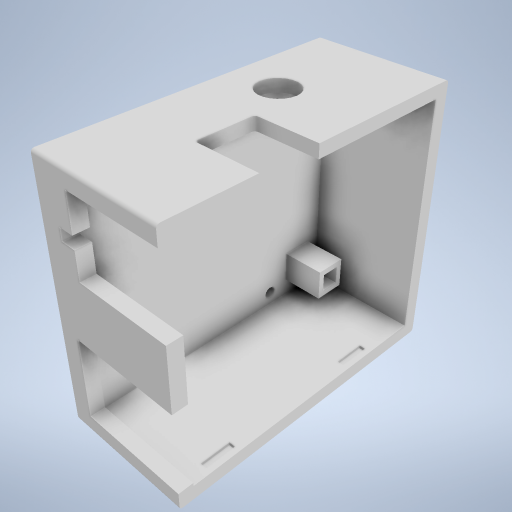
# Autodesk Inventor part: Enclosure_Top_v2
Saved by Autodesk Inventor 2023 (Build 270158030, 158C)
## iProperties
Created: 2023-12-07
Part Number: Enclosure_Top_v2
Material: Generic
Document SubType Name: Sheet Metal
Designer: Fabian
Density: 1 g/cm^3
Sheet Metal Rule: Default_mm
Appearance: Default
Author: Fabian
Autodesk Inventor part; units mm, degrees
ref_plane "YZ Plane" through (0, 0, 0) normal (1, 0, 0) x (0, 1, 0)
ref_plane "XZ Plane" through (0, 0, 0) normal (0, 1, 0) x (-1, 0, 0)
ref_plane "XY Plane" through (0, 0, 0) normal (0, 0, 1) x (1, 0, 0)
sketch "Sketch1" plane through (0, 0, 0) normal (1, 0, 0) x (0, 1, 0)
  line L0 (10.2141, 17.9541) -> (-31.7859, 17.9541)
  line L1 (-31.7859, 17.9541) -> (-31.7859, -30.1559)
  line L2 (-31.7859, -30.1559) -> (10.2141, -30.1559)
  line L3 (10.2141, -30.1559) -> (10.2141, 17.9541)
  point P0 (0, 0)
  dimension "d0" = 42
  dimension "d1" = 48.11
  constraints: 8 end point, 2 parallel, 1 horizontal, 1 perpendicular
  measures "d0" distance of L2.end L1.end
  measures "d1" distance of L1.end L0.end
extrude "BasePlate" add sketch "Sketch1" along normal blind 3
sketch "Sketch2" plane through (3, 0, 0) normal (1, 0, 0) x (0, 0, -1)
  point P0 (0, 0)
sketch "Sketch3" plane through (3, 0, 0) normal (1, 0, 0) x (0, 0, -1)
  line L0 (30.1559, 10.2141) -> (-17.9541, 10.2141) projected
  line L1 (-17.9541, -31.7859) -> (30.1559, -31.7859) projected
  line L2 (-17.9541, 10.2141) -> (30.1559, 10.2141)
  line L3 (30.1559, 10.2141) -> (30.1559, -31.7859)
  line L4 (30.1559, -31.7859) -> (-17.9541, -31.7859)
  line L5 (-17.9541, -31.7859) -> (-17.9541, 10.2141)
  line L6 (-15.5541, 8.2141) -> (27.7559, 8.2141)
  line L7 (27.7559, 8.2141) -> (27.7559, -29.3859)
  line L8 (27.7559, -29.3859) -> (-15.5541, -29.3859)
  line L9 (-15.5541, -29.3859) -> (-15.5541, 8.2141)
  point P0 (0, 0)
  point P1 (-17.9541, -10.7859)
  dimension "d4" = 2
  dimension "d5" = 2.4
  dimension "d6" = 2.4
  dimension "d7" = 2.4
  constraints: 16 end point, 4 parallel, 2 horizontal, 2 perpendicular, 1 midpoint
  measures "d4" distance between parallel lines of L0 L6
  measures "d5" distance between parallel lines of L1 L8
  measures "d6" distance from line of point (-17.954, -10.786) L9
  measures "d7" distance between parallel lines of L3 L7
extrude "Walls" add sketch "Sketch3" along normal blind 18.5
sketch "Sketch4" plane through (21.5, 0, 0) normal (1, 0, 0) x (0, 0, -1)
  line L0 (30.1559, 10.2141) -> (-17.9541, 10.2141) projected
  line L1 (-15.5541, 8.2141) -> (27.7559, 8.2141) projected
  line L2 (-4.1541, 10.2141) -> (5.2459, 10.2141)
  line L3 (5.2459, 10.2141) -> (5.2459, 8.2141)
  line L4 (5.2459, 8.2141) -> (-4.1541, 8.2141)
  line L5 (-4.1541, 8.2141) -> (-4.1541, 10.2141)
  line L6 (-17.9541, 10.2141) -> (-17.9541, -31.7859) projected
  point P0 (0, 0)
  point P1 (-4.1541, 9.2141)
  point P2 (5.2459, 10.2141)
  dimension "d10" = 9.4
  dimension "d11" = 13.8
  constraints: 8 end point, 2 parallel, 2 point on line, 1 horizontal, 1 midpoint, 1 perpendicular
  measures "d10" distance of L3.end L4.end
  measures "d11" distance from line of point (-4.154, 9.214) L6
extrude "USB-C" cut sketch "Sketch4" against normal blind 10.1
sketch "Sketch5" plane through (21.5, 0, 0) normal (1, 0, 0) x (0, 0, -1)
  line L0 (-17.9541, 10.2141) -> (-17.9541, -31.7859) projected
  line L1 (-15.5541, -29.3859) -> (-15.5541, 8.2141) projected
  line L2 (-17.9541, -4.8859) -> (-15.5541, -4.8859)
  line L3 (-15.5541, -4.8859) -> (-15.5541, 7.5141)
  line L4 (-15.5541, 7.5141) -> (-17.9541, 7.5141)
  line L5 (-17.9541, 7.5141) -> (-17.9541, -4.8859)
  line L6 (-4.1541, 10.2141) -> (-17.9541, 10.2141) projected
  point P0 (0, 0)
  point P1 (-16.7541, 7.5141)
  point P2 (-17.9541, 7.5141)
  point P3 (-15.5541, -4.8859)
  dimension "d14" = 12.4
  dimension "d15" = 2.7
  constraints: 8 end point, 2 parallel, 2 point on line, 1 horizontal, 1 midpoint, 1 perpendicular
  measures "d14" distance of L3.end L2.end
  measures "d15" distance from line of L6 point (-16.754, 7.514)
extrude "PowerConnector1" cut sketch "Sketch5" against normal blind 15.5
sketch "Sketch6" plane through (6, 0, 0) normal (1, 0, 0) x (0, 0, -1)
  line L0 (-17.9541, 10.2141) -> (-17.9541, -31.7859) projected
  line L1 (-17.9541, -0.3859) -> (-15.5541, -0.3859)
  line L2 (-15.5541, -0.3859) -> (-15.5541, 1.6141)
  line L3 (-15.5541, 1.6141) -> (-17.9541, 1.6141)
  line L4 (-17.9541, 1.6141) -> (-17.9541, -0.3859)
  line L5 (-17.9541, 7.5141) -> (-15.5541, 7.5141) projected
  point P0 (0, 0)
  dimension "d18" = 2.4
  dimension "d19" = 2
  dimension "d20" = 5.9
  constraints: 8 end point, 2 parallel, 1 horizontal, 1 perpendicular, 1 point on line
  measures "d18" distance of L3.end L2.end
  measures "d19" distance of L1.end L2.end
  measures "d20" distance between parallel lines of L5 L3
extrude "PowerConnector2" cut sketch "Sketch6" against normal blind 2.5
sketch "Sketch8" plane through (21.5, 0, 0) normal (1, 0, 0) x (0, 0, -1)
  line L0 (-17.9541, 10.2141) -> (-17.9541, -31.7859) projected
  line L1 (-15.5541, 8.2141) -> (-15.5541, -29.3859) projected
  line L2 (-17.9541, -28.7859) -> (-15.5541, -28.7859)
  line L3 (-15.5541, -28.7859) -> (-15.5541, -15.1859)
  line L4 (-15.5541, -15.1859) -> (-17.9541, -15.1859)
  line L5 (-17.9541, -15.1859) -> (-17.9541, -28.7859)
  line L6 (-17.9541, -31.7859) -> (30.1559, -31.7859) projected
  point P0 (0, 0)
  dimension "d23" = 13.6
  dimension "d24" = 3
  constraints: 8 end point, 2 parallel, 2 point on line, 1 horizontal, 1 perpendicular
  measures "d23" distance of L3.end L2.end
  measures "d24" distance between parallel lines of L6 L2
extrude "RJ-12" cut sketch "Sketch8" against normal blind 18.1
fillet "Fillet1" radius 0.5 4 edges at (10.75, 10.2141, 17.9541) (10.75, -31.7859, 17.9541) (10.75, 10.2141, -30.1559) (10.75, -31.7859, -30.1559)
sketch "Sketch9" plane through (0, 0, 0) normal (-1, 0, 0) x (0, 0, 1)
  line L0 (-24.5559, -25.4859) -> (-21.5559, -25.4859)
  line L1 (-21.5559, -25.4859) -> (-21.5559, -22.4859)
  line L2 (-21.5559, -22.4859) -> (-24.5559, -22.4859)
  line L3 (-24.5559, -22.4859) -> (-24.5559, -25.4859)
  line L4 (-30.1559, -31.2859) -> (-30.1559, 9.7141) projected
  line L5 (17.4541, -31.7859) -> (-29.6559, -31.7859) projected
  point P0 (0, 0)
  point P1 (-24.5559, -23.9859)
  dimension "d28" = 3
  dimension "d29" = 3
  dimension "d30" = 5.6
  dimension "d31" = 6.3
  constraints: 8 end point, 2 parallel, 1 horizontal, 1 midpoint, 1 perpendicular
  measures "d28" distance of L2.end L1.end
  measures "d29" distance of L1.end L0.end
  measures "d30" distance from line of L4 point (-24.556, -23.986)
  measures "d31" distance between parallel lines of L5 L0
extrude "ZBButton" cut sketch "Sketch9" against normal blind 3
sketch "Sketch10" plane through (0, 0, 0) normal (-1, 0, 0) x (0, 0, 1)
  line L0 (-24.5559, 0.9141) -> (-21.5559, 0.9141)
  line L1 (-21.5559, 0.9141) -> (-21.5559, 3.9141)
  line L2 (-21.5559, 3.9141) -> (-24.5559, 3.9141)
  line L3 (-24.5559, 3.9141) -> (-24.5559, 0.9141)
  line L4 (-30.1559, -31.2859) -> (-30.1559, 9.7141) projected
  line L5 (-29.6559, 10.2141) -> (17.4541, 10.2141) projected
  point P0 (0, 0)
  point P1 (-24.5559, 2.4141)
  dimension "d34" = 3
  dimension "d35" = 3
  dimension "d36" = 5.6
  dimension "d37" = 6.3
  constraints: 8 end point, 2 parallel, 1 horizontal, 1 midpoint, 1 perpendicular
  measures "d34" distance of L2.end L1.end
  measures "d35" distance of L1.end L0.end
  measures "d36" distance from line of L4 point (-24.556, 2.414)
  measures "d37" distance between parallel lines of L5 L2
extrude "ResetButton" cut sketch "Sketch10" against normal blind 3
sketch "Sketch11" plane through (3, 0, 0) normal (1, 0, 0) x (0, 0, -1)
  line L0 (25.5559, 4.9141) -> (20.5559, 4.9141)
  line L1 (20.5559, 4.9141) -> (20.5559, -0.0859)
  line L2 (20.5559, -0.0859) -> (25.5559, -0.0859)
  line L3 (25.5559, -0.0859) -> (25.5559, 4.9141)
  line L4 (21.5559, 3.9141) -> (24.5559, 3.9141) projected
  line L5 (24.5559, 3.9141) -> (24.5559, 0.9141) projected
  line L6 (25.5559, -21.4859) -> (20.5559, -21.4859)
  line L7 (20.5559, -21.4859) -> (20.5559, -26.4859)
  line L8 (20.5559, -26.4859) -> (25.5559, -26.4859)
  line L9 (25.5559, -26.4859) -> (25.5559, -21.4859)
  line L10 (24.5559, -22.4859) -> (24.5559, -25.4859) projected
  line L11 (21.5559, -22.4859) -> (24.5559, -22.4859) projected
  line L12 (24.5559, 0.9141) -> (21.5559, 0.9141) projected
  line L13 (24.5559, 3.9141) -> (21.5559, 3.9141)
  line L14 (21.5559, 3.9141) -> (21.5559, 0.9141)
  line L15 (21.5559, 0.9141) -> (24.5559, 0.9141)
  line L16 (24.5559, 0.9141) -> (24.5559, 3.9141)
  line L17 (21.5559, -25.4859) -> (21.5559, -22.4859) projected
  line L18 (24.5559, -22.4859) -> (21.5559, -22.4859)
  line L19 (21.5559, -22.4859) -> (21.5559, -25.4859)
  line L20 (21.5559, -25.4859) -> (24.5559, -25.4859)
  line L21 (24.5559, -25.4859) -> (24.5559, -22.4859)
  point P0 (0, 0)
  point P1 (23.0559, -22.4859)
  dimension "d40" = 5
  dimension "d41" = 5
  dimension "d42" = 1
  dimension "d43" = 1
  dimension "d44" = 5
  dimension "d45" = 5
  dimension "d46" = 1
  dimension "d47" = 1
  constraints: 32 end point, 8 parallel, 4 horizontal, 4 perpendicular, 1 midpoint
  measures "d40" distance of L2.end L1.end
  measures "d41" distance of L1.end L0.end
  measures "d42" distance between parallel lines of L4 L0
  measures "d43" distance between parallel lines of L3 L5
  measures "d44" distance of L8.end L7.end
  measures "d45" distance of L7.end L6.end
  measures "d46" distance between parallel lines of L9 L10
  measures "d47" distance from line of point (23.056, -22.486) L6
extrude "ButtonFuehrung" add sketch "Sketch11" along normal blind 7
sketch "Sketch12" plane through (0, 0, 0) normal (-1, 0, 0) x (0, 0, 1)
  circle A0 centre (-16.9559, -27.1859) radius 1
  line L0 (17.4541, -31.7859) -> (-29.6559, -31.7859) projected
  line L1 (-30.1559, -31.2859) -> (-30.1559, 9.7141) projected
  point P0 (0, 0)
  dimension "d50" = 2
  dimension "d51" = 4.6
  dimension "d52" = 13.2
  constraints: 1 centre point
  measures "d50" diameter of A0
  measures "d51" distance from line of L0 A0.centre
  measures "d52" distance from line of L1 A0.centre
extrude "LED" cut sketch "Sketch12" against normal blind 3
sketch "Sketch13" plane through (11.4, 10.2141, 4.1541) normal (0, 1, 0) x (1, 0, 0)
  circle A0 centre (-3.4, 16.91) radius 3.2
  line L0 (-11.4, 33.81) -> (-11.4, -13.3) projected
  line L1 (10.1, 34.31) -> (-11.4, 34.31) projected
  point P0 (-11.4, 4.1541)
  dimension "d55" = 6.4
  dimension "d56" = 8
  dimension "d57" = 17.4
  constraints: 1 centre point
  measures "d55" diameter of A0
  measures "d56" distance from line of L0 A0.centre
  measures "d57" distance from line of L1 A0.centre
extrude "Antenna" cut sketch "Sketch13" against normal blind 2
sketch "Sketch14" plane through (3, 8.2141, -27.7559) normal (0, -1, 0) x (1, 0, 0)
  line L0 (17.5, 40.31) -> (16.5, 40.31)
  line L1 (16.5, 40.31) -> (16.5, 35.31)
  line L2 (16.5, 35.31) -> (17.5, 35.31)
  line L3 (17.5, 35.31) -> (17.5, 40.31)
  line L4 (18.5, 43.31) -> (18.5, 31.91) projected
  point P0 (-3, 27.7559)
  point P1 (17.5, 37.81)
  dimension "d60" = 1
  dimension "d61" = 5
  dimension "d62" = 1
  dimension "d63" = 5.5
  constraints: 8 end point, 2 parallel, 1 horizontal, 1 midpoint, 1 perpendicular
  measures "d60" distance of L2.end L1.end
  measures "d61" distance of L1.end L0.end
  measures "d62" distance between parallel lines of L4 L3
  measures "d63" vertical distance of L4.start point (17.5, 37.81)
extrude "Extrusion12" cut sketch "Sketch14" against normal blind 0.5
sketch "Sketch15" plane through (3, 8.2141, -27.7559) normal (0, -1, 0) x (1, 0, 0)
  line L0 (17.5, 13.5) -> (16.5, 13.5)
  line L1 (16.5, 13.5) -> (16.5, 8.5)
  line L2 (16.5, 8.5) -> (17.5, 8.5)
  line L3 (17.5, 8.5) -> (17.5, 13.5)
  line L4 (18.5, 22.51) -> (18.5, 0) projected
  line L5 (0, 0) -> (18.5, 0) projected
  point P0 (-3, 27.7559)
  point P1 (17.5, 11)
  dimension "d66" = 1
  dimension "d67" = 5
  dimension "d68" = 1
  dimension "d69" = 11
  constraints: 8 end point, 2 parallel, 1 horizontal, 1 midpoint, 1 perpendicular
  measures "d66" distance of L2.end L1.end
  measures "d67" distance of L1.end L0.end
  measures "d68" distance from line of L4 point (17.5, 11)
  measures "d69" distance from line of L5 point (17.5, 11)
extrude "Extrusion13" cut sketch "Sketch15" against normal blind 0.5
sketch "Sketch16" plane through (3, -29.3859, 15.5541) normal (0, 1, 0) x (1, 0, 0)
  line L0 (17.5, 8) -> (16.5, 8)
  line L1 (16.5, 8) -> (16.5, 3)
  line L2 (16.5, 3) -> (17.5, 3)
  line L3 (17.5, 3) -> (17.5, 8)
  line L4 (18.5, 43.31) -> (18.5, 0) projected
  line L5 (0, 0) -> (18.5, 0) projected
  point P0 (-3, 15.5541)
  point P1 (17.5, 5.5)
  dimension "d72" = 1
  dimension "d73" = 5
  dimension "d74" = 1
  dimension "d75" = 5.5
  constraints: 8 end point, 2 parallel, 1 horizontal, 1 midpoint, 1 perpendicular
  measures "d72" distance of L2.end L1.end
  measures "d73" distance of L1.end L0.end
  measures "d74" distance between parallel lines of L4 L3
  measures "d75" distance from line of L5 point (17.5, 5.5)
extrude "Extrusion14" cut sketch "Sketch16" against normal blind 0.5
sketch "Sketch17" plane through (3, -29.3859, 15.5541) normal (0, 1, 0) x (1, 0, 0)
  line L0 (17.5, 34.81) -> (16.5, 34.81)
  line L1 (16.5, 34.81) -> (16.5, 29.81)
  line L2 (16.5, 29.81) -> (17.5, 29.81)
  line L3 (17.5, 29.81) -> (17.5, 34.81)
  line L4 (18.5, 43.31) -> (18.5, 0) projected
  line L5 (0, 43.31) -> (18.5, 43.31) projected
  point P0 (-3, 15.5541)
  point P1 (17.5, 32.31)
  dimension "d78" = 1
  dimension "d79" = 5
  dimension "d80" = 1
  dimension "d81" = 11
  constraints: 8 end point, 2 parallel, 1 horizontal, 1 midpoint, 1 perpendicular
  measures "d78" distance of L2.end L1.end
  measures "d79" distance of L1.end L0.end
  measures "d80" distance between parallel lines of L4 L3
  measures "d81" distance from line of L5 point (17.5, 32.31)
extrude "Extrusion15" cut sketch "Sketch17" against normal blind 0.5
fillet "Fillet2" radius 0.5 2 edges at (11.4, 9.2141, -5.2459) (11.4, 9.2141, 4.1541)
sketch "Sketch18" plane through (0, 0, 0) normal (-1, 0, 0) x (0, 0, 1)
  line L0 (-24.8059, 9.0246) -> (-24.8059, -4.4756) construction
  line L1 (-24.8059, -4.4756) -> (-28.9977, -4.4756) construction
  line L2 (-28.9977, -4.4756) -> (-28.9977, 9.0246) construction
  line L3 (-28.9977, 9.0246) -> (-24.8059, 9.0246) construction
  line L4 (-24.8059, -15.1002) -> (-24.8059, -31.4737) construction
  line L5 (-24.8059, -31.4737) -> (-30.0114, -31.4737) construction
  line L6 (-30.0114, -31.4737) -> (-30.0114, -15.1002) construction
  line L7 (-30.0114, -15.1002) -> (-24.8059, -15.1002) construction
  line L8 (-24.5559, -25.4859) -> (-24.5559, -22.4859) projected
  line L9 (-24.5559, 0.9141) -> (-24.5559, 3.9141) projected
  line L10 (-28.8059, 5.5238) -> (-28.8059, 6.2142)
  line L11 (-28.8059, 6.2142) -> (-27.2144, 7.4784)
  line L12 (-27.2144, 7.4784) -> (-27.2144, 8.0878)
  line L13 (-27.2144, 8.0878) -> (-28.8059, 8.0878)
  line L14 (-28.8059, 8.0878) -> (-28.8059, 8.6194)
  line L15 (-28.8059, 8.6194) -> (-24.8059, 8.6194)
  line L16 (-24.8059, 8.6194) -> (-24.8059, 7.5886)
  spline S0 degree 2 poles (-24.8059, 7.5886) (-24.8059, 7.245) (-24.8805, 6.7815) (-25.0166, 6.5708) knots 0 0 0 1 2 2 2
  spline S1 degree 2 poles (-25.0166, 6.5708) (-25.1528, 6.3601) (-25.5774, 6.117) (-25.8918, 6.117) knots 0 0 0 1 2 2 2
  spline S2 degree 2 poles (-25.8918, 6.117) (-26.3294, 6.117) (-26.9226, 6.5643) (-27.0653, 6.9468) knots 0 0 0 1 2 2 2
  line L17 (-27.0653, 6.9468) -> (-28.8059, 5.5238)
  spline S3 degree 2 poles (-25.934, 6.6713) (-25.7589, 6.6713) (-25.4899, 6.7944) (-25.4024, 6.9241) knots 0 0 0 1 2 2 2
  spline S4 degree 2 poles (-25.4024, 6.9241) (-25.3278, 7.0375) (-25.2662, 7.339) (-25.2662, 7.5594) knots 0 0 0 1 2 2 2
  line L18 (-25.2662, 7.5594) -> (-25.2662, 8.0878)
  line L19 (-25.2662, 8.0878) -> (-26.7703, 8.0878)
  line L20 (-26.7703, 8.0878) -> (-26.7703, 7.621)
  spline S5 degree 2 poles (-26.7703, 7.621) (-26.7703, 7.3909) (-26.6892, 7.0246) (-26.5628, 6.8982) knots 0 0 0 1 2 2 2
  spline S6 degree 2 poles (-26.5628, 6.8982) (-26.4526, 6.7815) (-26.1414, 6.6713) (-25.934, 6.6713) knots 0 0 0 1 2 2 2
  spline S7 degree 2 poles (-28.874, 3.9419) (-28.874, 4.6615) (-28.0669, 5.4525) (-27.3213, 5.4525) knots 0 0 0 1 2 2 2
  spline S8 degree 2 poles (-27.3213, 5.4525) (-26.5888, 5.4525) (-25.72, 4.6842) (-25.72, 4.0651) knots 0 0 0 1 2 2 2
  spline S9 degree 2 poles (-25.72, 4.0651) (-25.72, 3.7863) (-25.8821, 3.3552) (-26.0539, 3.1964) knots 0 0 0 1 2 2 2
  spline S10 degree 2 poles (-26.0539, 3.1964) (-26.2257, 3.0343) (-26.7217, 2.8625) (-27.0815, 2.8625) knots 0 0 0 1 2 2 2
  line L21 (-27.0815, 2.8625) -> (-27.357, 2.8625)
  line L22 (-27.357, 2.8625) -> (-27.357, 4.9403)
  spline S11 degree 2 poles (-27.357, 4.9403) (-27.8789, 4.9403) (-28.4332, 4.4152) (-28.4332, 3.9484) knots 0 0 0 1 2 2 2
  spline S12 degree 2 poles (-28.4332, 3.9484) (-28.4332, 3.7831) (-28.3586, 3.4622) (-28.3003, 3.3325) knots 0 0 0 1 2 2 2
  spline S13 degree 2 poles (-28.3003, 3.3325) (-28.2354, 3.1964) (-28.122, 3.0084) (-28.0701, 2.9468) knots 0 0 0 1 2 2 2
  line L23 (-28.0701, 2.9468) -> (-28.0701, 2.9176)
  line L24 (-28.0701, 2.9176) -> (-28.6212, 2.9176)
  spline S14 degree 2 poles (-28.6212, 2.9176) (-28.6568, 3.0051) (-28.7606, 3.2709) (-28.7897, 3.3747) knots 0 0 0 1 2 2 2
  spline S15 degree 2 poles (-28.7897, 3.3747) (-28.8319, 3.5205) (-28.874, 3.7604) (-28.874, 3.9419) knots 0 0 0 1 2 2 2
  spline S16 degree 2 poles (-26.9713, 3.3552) (-26.767, 3.3617) (-26.4688, 3.446) (-26.3683, 3.527) knots 0 0 0 1 2 2 2
  spline S17 degree 2 poles (-26.3683, 3.527) (-26.2549, 3.6145) (-26.135, 3.8901) (-26.135, 4.0943) knots 0 0 0 1 2 2 2
  spline S18 degree 2 poles (-26.135, 4.0943) (-26.135, 4.2952) (-26.2549, 4.5772) (-26.3716, 4.6939) knots 0 0 0 1 2 2 2
  spline S19 degree 2 poles (-26.3716, 4.6939) (-26.4915, 4.8074) (-26.78, 4.9241) (-26.9713, 4.9403) knots 0 0 0 1 2 2 2
  line L25 (-26.9713, 4.9403) -> (-26.9713, 3.3552)
  spline S20 degree 2 poles (-28.8773, 1.54) (-28.8773, 1.8414) (-28.7152, 2.3633) (-28.6244, 2.5351) knots 0 0 0 1 2 2 2
  line L26 (-28.6244, 2.5351) -> (-28.0572, 2.5351)
  line L27 (-28.0572, 2.5351) -> (-28.0572, 2.5092)
  spline S21 degree 2 poles (-28.0572, 2.5092) (-28.109, 2.4443) (-28.2322, 2.2693) (-28.3003, 2.1234) knots 0 0 0 1 2 2 2
  spline S22 degree 2 poles (-28.3003, 2.1234) (-28.3619, 1.997) (-28.4526, 1.6858) (-28.4526, 1.5205) knots 0 0 0 1 2 2 2
  spline S23 degree 2 poles (-28.4526, 1.5205) (-28.4526, 1.4006) (-28.3975, 1.1251) (-28.3521, 1.0602) knots 0 0 0 1 2 2 2
  spline S24 degree 2 poles (-28.3521, 1.0602) (-28.2905, 0.9662) (-28.1512, 0.8819) (-28.0085, 0.8819) knots 0 0 0 1 2 2 2
  spline S25 degree 2 poles (-28.0085, 0.8819) (-27.8303, 0.8819) (-27.6455, 1.0764) (-27.5839, 1.326) knots 0 0 0 1 2 2 2
  spline S26 degree 2 poles (-27.5839, 1.326) (-27.5612, 1.4233) (-27.4964, 1.7345) (-27.4607, 1.8674) knots 0 0 0 1 2 2 2
  spline S27 degree 2 poles (-27.4607, 1.8674) (-27.3602, 2.211) (-26.9453, 2.5221) (-26.6503, 2.5221) knots 0 0 0 1 2 2 2
  spline S28 degree 2 poles (-26.6503, 2.5221) (-26.2419, 2.5221) (-25.733, 1.9095) (-25.733, 1.4038) knots 0 0 0 1 2 2 2
  spline S29 degree 2 poles (-25.733, 1.4038) (-25.733, 1.1542) (-25.8562, 0.6486) (-25.9502, 0.4768) knots 0 0 0 1 2 2 2
  line L28 (-25.9502, 0.4768) -> (-26.4915, 0.4768)
  line L29 (-26.4915, 0.4768) -> (-26.4915, 0.5027)
  spline S30 degree 2 poles (-26.4915, 0.5027) (-26.3359, 0.6972) (-26.1576, 1.1704) (-26.1576, 1.4136) knots 0 0 0 1 2 2 2
  spline S31 degree 2 poles (-26.1576, 1.4136) (-26.1576, 1.6631) (-26.3683, 2.0067) (-26.579, 2.0067) knots 0 0 0 1 2 2 2
  spline S32 degree 2 poles (-26.579, 2.0067) (-26.7703, 2.0067) (-26.955, 1.8025) (-27.0134, 1.5756) knots 0 0 0 1 2 2 2
  spline S33 degree 2 poles (-27.0134, 1.5756) (-27.0426, 1.4654) (-27.1009, 1.1867) (-27.1366, 1.0343) knots 0 0 0 1 2 2 2
  spline S34 degree 2 poles (-27.1366, 1.0343) (-27.2209, 0.7037) (-27.6066, 0.3666) (-27.9405, 0.3666) knots 0 0 0 1 2 2 2
  spline S35 degree 2 poles (-27.9405, 0.3666) (-28.135, 0.3666) (-28.4786, 0.5189) (-28.605, 0.668) knots 0 0 0 1 2 2 2
  spline S36 degree 2 poles (-28.605, 0.668) (-28.7379, 0.8268) (-28.8773, 1.232) (-28.8773, 1.54) knots 0 0 0 1 2 2 2
  spline S37 degree 2 poles (-28.874, -1.4065) (-28.874, -0.6869) (-28.0669, 0.104) (-27.3213, 0.104) knots 0 0 0 1 2 2 2
  spline S38 degree 2 poles (-27.3213, 0.104) (-26.5888, 0.104) (-25.72, -0.6642) (-25.72, -1.2834) knots 0 0 0 1 2 2 2
  spline S39 degree 2 poles (-25.72, -1.2834) (-25.72, -1.5621) (-25.8821, -1.9933) (-26.0539, -2.1521) knots 0 0 0 1 2 2 2
  spline S40 degree 2 poles (-26.0539, -2.1521) (-26.2257, -2.3142) (-26.7217, -2.486) (-27.0815, -2.486) knots 0 0 0 1 2 2 2
  line L30 (-27.0815, -2.486) -> (-27.357, -2.486)
  line L31 (-27.357, -2.486) -> (-27.357, -0.4082)
  spline S41 degree 2 poles (-27.357, -0.4082) (-27.8789, -0.4082) (-28.4332, -0.9333) (-28.4332, -1.4001) knots 0 0 0 1 2 2 2
  spline S42 degree 2 poles (-28.4332, -1.4001) (-28.4332, -1.5654) (-28.3586, -1.8863) (-28.3003, -2.0159) knots 0 0 0 1 2 2 2
  spline S43 degree 2 poles (-28.3003, -2.0159) (-28.2354, -2.1521) (-28.122, -2.3401) (-28.0701, -2.4017) knots 0 0 0 1 2 2 2
  line L32 (-28.0701, -2.4017) -> (-28.0701, -2.4309)
  line L33 (-28.0701, -2.4309) -> (-28.6212, -2.4309)
  spline S44 degree 2 poles (-28.6212, -2.4309) (-28.6568, -2.3433) (-28.7606, -2.0775) (-28.7897, -1.9738) knots 0 0 0 1 2 2 2
  spline S45 degree 2 poles (-28.7897, -1.9738) (-28.8319, -1.8279) (-28.874, -1.5881) (-28.874, -1.4065) knots 0 0 0 1 2 2 2
  spline S46 degree 2 poles (-26.9713, -1.9933) (-26.767, -1.9868) (-26.4688, -1.9025) (-26.3683, -1.8215) knots 0 0 0 1 2 2 2
  spline S47 degree 2 poles (-26.3683, -1.8215) (-26.2549, -1.7339) (-26.135, -1.4584) (-26.135, -1.2542) knots 0 0 0 1 2 2 2
  spline S48 degree 2 poles (-26.135, -1.2542) (-26.135, -1.0532) (-26.2549, -0.7712) (-26.3716, -0.6545) knots 0 0 0 1 2 2 2
  spline S49 degree 2 poles (-26.3716, -0.6545) (-26.4915, -0.5411) (-26.78, -0.4244) (-26.9713, -0.4082) knots 0 0 0 1 2 2 2
  line L34 (-26.9713, -0.4082) -> (-26.9713, -1.9933)
  spline S50 degree 2 poles (-28.8643, -3.9057) (-28.8643, -3.4941) (-28.3943, -3.0305) (-27.8854, -3.0305) knots 0 0 0 1 2 2 2
  line L35 (-27.8854, -3.0305) -> (-26.2225, -3.0305)
  line L36 (-26.2225, -3.0305) -> (-26.2225, -2.6902)
  line L37 (-26.2225, -2.6902) -> (-25.8043, -2.6902)
  line L38 (-25.8043, -2.6902) -> (-25.8043, -3.0305)
  line L39 (-25.8043, -3.0305) -> (-24.9421, -3.0305)
  line L40 (-24.9421, -3.0305) -> (-24.9421, -3.5362)
  line L41 (-24.9421, -3.5362) -> (-25.8043, -3.5362)
  line L42 (-25.8043, -3.5362) -> (-25.8043, -4.4665)
  line L43 (-25.8043, -4.4665) -> (-26.2225, -4.4665)
  line L44 (-26.2225, -4.4665) -> (-26.2225, -3.5362)
  line L45 (-26.2225, -3.5362) -> (-27.652, -3.5362)
  spline S51 degree 2 poles (-27.652, -3.5362) (-27.8789, -3.5362) (-28.1285, -3.5524) (-28.2354, -3.6075) knots 0 0 0 1 2 2 2
  spline S52 degree 2 poles (-28.2354, -3.6075) (-28.3294, -3.6529) (-28.4234, -3.8571) (-28.4234, -4.0322) knots 0 0 0 1 2 2 2
  spline S53 degree 2 poles (-28.4234, -4.0322) (-28.4234, -4.1553) (-28.3489, -4.3855) (-28.3262, -4.4373) knots 0 0 0 1 2 2 2
  line L46 (-28.3262, -4.4373) -> (-28.3262, -4.4665)
  line L47 (-28.3262, -4.4665) -> (-28.78, -4.4665)
  spline S54 degree 2 poles (-28.78, -4.4665) (-28.8189, -4.3239) (-28.8643, -4.0322) (-28.8643, -3.9057) knots 0 0 0 1 2 2 2
  line L48 (-28.8319, -18.0564) -> (-28.8319, -15.2623)
  line L49 (-28.8319, -15.2623) -> (-28.3359, -15.2623)
  line L50 (-28.3359, -15.2623) -> (-25.3051, -17.4016)
  line L51 (-25.3051, -17.4016) -> (-25.3051, -15.3595)
  line L52 (-25.3051, -15.3595) -> (-24.8319, -15.3595)
  line L53 (-24.8319, -15.3595) -> (-24.8319, -18.0013)
  line L54 (-24.8319, -18.0013) -> (-25.3116, -18.0013)
  line L55 (-25.3116, -18.0013) -> (-28.3586, -15.8392)
  line L56 (-28.3586, -15.8392) -> (-28.3586, -18.0564)
  line L57 (-28.3586, -18.0564) -> (-28.8319, -18.0564)
  line L58 (-28.8319, -19.058) -> (-28.8319, -18.5524)
  line L59 (-28.8319, -18.5524) -> (-25.8303, -18.5524)
  line L60 (-25.8303, -18.5524) -> (-25.8303, -19.058)
  line L61 (-25.8303, -19.058) -> (-28.8319, -19.058)
  line L62 (-25.3311, -19.0937) -> (-25.3311, -18.52)
  line L63 (-25.3311, -18.52) -> (-24.8059, -18.52)
  line L64 (-24.8059, -18.52) -> (-24.8059, -19.0937)
  line L65 (-24.8059, -19.0937) -> (-25.3311, -19.0937)
  spline S55 degree 2 poles (-29.3116, -19.9073) (-29.3343, -19.9592) (-29.4056, -20.1569) (-29.4348, -20.2833) knots 0 0 0 1 2 2 2
  spline S56 degree 2 poles (-29.4348, -20.2833) (-29.4704, -20.4227) (-29.5126, -20.6593) (-29.5126, -20.7987) knots 0 0 0 1 2 2 2
  spline S57 degree 2 poles (-29.5126, -20.7987) (-29.5126, -21.0321) (-29.3894, -21.3563) (-29.2792, -21.447) knots 0 0 0 1 2 2 2
  spline S58 degree 2 poles (-29.2792, -21.447) (-29.169, -21.5345) (-28.8805, -21.6026) (-28.6957, -21.6026) knots 0 0 0 1 2 2 2
  line L66 (-28.6957, -21.6026) -> (-28.4332, -21.6026)
  spline S59 degree 2 poles (-28.4332, -21.6026) (-28.6115, -21.3984) (-28.78, -21.0062) (-28.78, -20.7112) knots 0 0 0 1 2 2 2
  spline S60 degree 2 poles (-28.78, -20.7112) (-28.78, -20.1991) (-28.0183, -19.5929) (-27.3019, -19.5929) knots 0 0 0 1 2 2 2
  spline S61 degree 2 poles (-27.3019, -19.5929) (-26.9291, -19.5929) (-26.3521, -19.8036) (-26.1479, -19.9786) knots 0 0 0 1 2 2 2
  spline S62 degree 2 poles (-26.1479, -19.9786) (-25.9567, -20.1472) (-25.746, -20.6107) (-25.746, -20.8571) knots 0 0 0 1 2 2 2
  spline S63 degree 2 poles (-25.746, -20.8571) (-25.746, -21.0905) (-25.8562, -21.4308) (-25.9567, -21.6026) knots 0 0 0 1 2 2 2
  line L67 (-25.9567, -21.6026) -> (-25.8303, -21.6318)
  line L68 (-25.8303, -21.6318) -> (-25.8303, -22.1083)
  line L69 (-25.8303, -22.1083) -> (-28.4883, -22.1083)
  spline S64 degree 2 poles (-28.4883, -22.1083) (-29.2533, -22.1083) (-29.9664, -21.4438) (-29.9664, -20.7598) knots 0 0 0 1 2 2 2
  spline S65 degree 2 poles (-29.9664, -20.7598) (-29.9664, -20.5394) (-29.8951, -20.0791) (-29.8367, -19.8814) knots 0 0 0 1 2 2 2
  line L70 (-29.8367, -19.8814) -> (-29.3116, -19.8814)
  line L71 (-29.3116, -19.8814) -> (-29.3116, -19.9073)
  line L72 (-28.0183, -21.6026) -> (-26.3683, -21.6026)
  spline S66 degree 2 poles (-26.3683, -21.6026) (-26.2776, -21.4146) (-26.1998, -21.0969) (-26.1998, -20.9381) knots 0 0 0 1 2 2 2
  spline S67 degree 2 poles (-26.1998, -20.9381) (-26.1998, -20.5556) (-26.7638, -20.1148) (-27.2922, -20.1148) knots 0 0 0 1 2 2 2
  spline S68 degree 2 poles (-27.2922, -20.1148) (-27.7914, -20.1148) (-28.3132, -20.4486) (-28.3132, -20.8247) knots 0 0 0 1 2 2 2
  spline S69 degree 2 poles (-28.3132, -20.8247) (-28.3132, -21.0224) (-28.1576, -21.4373) (-28.0183, -21.6026) knots 0 0 0 1 2 2 2
  spline S70 degree 2 poles (-27.6033, -25.5929) (-27.9016, -25.5929) (-28.3586, -25.366) (-28.5077, -25.178) knots 0 0 0 1 2 2 2
  spline S71 degree 2 poles (-28.5077, -25.178) (-28.6828, -24.9511) (-28.8319, -24.4357) (-28.8319, -24.0273) knots 0 0 0 1 2 2 2
  line L73 (-28.8319, -24.0273) -> (-28.8319, -22.8798)
  line L74 (-28.8319, -22.8798) -> (-24.8319, -22.8798)
  line L75 (-24.8319, -22.8798) -> (-24.8319, -23.9397)
  spline S72 degree 2 poles (-24.8319, -23.9397) (-24.8319, -24.3676) (-24.887, -24.7955) (-24.9939, -24.99) knots 0 0 0 1 2 2 2
  spline S73 degree 2 poles (-24.9939, -24.99) (-25.1074, -25.2072) (-25.4802, -25.4049) (-25.733, -25.4049) knots 0 0 0 1 2 2 2
  spline S74 degree 2 poles (-25.733, -25.4049) (-26.015, -25.4049) (-26.4623, -25.1067) (-26.5888, -24.8441) knots 0 0 0 1 2 2 2
  line L76 (-26.5888, -24.8441) -> (-26.6082, -24.8441)
  spline S75 degree 2 poles (-26.6082, -24.8441) (-26.7055, -25.2007) (-27.2209, -25.5929) (-27.6033, -25.5929) knots 0 0 0 1 2 2 2
  spline S76 degree 2 poles (-27.626, -25.0386) (-27.3991, -25.0386) (-27.1074, -24.9089) (-27.0037, -24.7145) knots 0 0 0 1 2 2 2
  spline S77 degree 2 poles (-27.0037, -24.7145) (-26.9388, -24.588) (-26.8999, -24.2898) (-26.8999, -24.0143) knots 0 0 0 1 2 2 2
  line L77 (-26.8999, -24.0143) -> (-26.8999, -23.4114)
  line L78 (-26.8999, -23.4114) -> (-28.3781, -23.4114)
  line L79 (-28.3781, -23.4114) -> (-28.3781, -23.8425)
  spline S78 degree 2 poles (-28.3781, -23.8425) (-28.3781, -24.1926) (-28.3132, -24.5945) (-28.2095, -24.7501) knots 0 0 0 1 2 2 2
  spline S79 degree 2 poles (-28.2095, -24.7501) (-28.1025, -24.8992) (-27.8367, -25.0386) (-27.626, -25.0386) knots 0 0 0 1 2 2 2
  spline S80 degree 2 poles (-25.8076, -24.8506) (-25.6649, -24.8506) (-25.451, -24.7533) (-25.3894, -24.6464) knots 0 0 0 1 2 2 2
  spline S81 degree 2 poles (-25.3894, -24.6464) (-25.3181, -24.5167) (-25.2857, -24.2023) (-25.2857, -23.9203) knots 0 0 0 1 2 2 2
  line L80 (-25.2857, -23.9203) -> (-25.2857, -23.4114)
  line L81 (-25.2857, -23.4114) -> (-26.4559, -23.4114)
  line L82 (-26.4559, -23.4114) -> (-26.4559, -24.0143)
  spline S82 degree 2 poles (-26.4559, -24.0143) (-26.4559, -24.2639) (-26.404, -24.5005) (-26.323, -24.6269) knots 0 0 0 1 2 2 2
  spline S83 degree 2 poles (-26.323, -24.6269) (-26.2452, -24.7501) (-25.9956, -24.8506) (-25.8076, -24.8506) knots 0 0 0 1 2 2 2
  spline S84 degree 2 poles (-28.8999, -27.3854) (-28.8999, -26.6658) (-28.0928, -25.8749) (-27.3473, -25.8749) knots 0 0 0 1 2 2 2
  spline S85 degree 2 poles (-27.3473, -25.8749) (-26.6147, -25.8749) (-25.746, -26.6431) (-25.746, -27.2623) knots 0 0 0 1 2 2 2
  spline S86 degree 2 poles (-25.746, -27.2623) (-25.746, -27.541) (-25.908, -27.9722) (-26.0798, -28.131) knots 0 0 0 1 2 2 2
  spline S87 degree 2 poles (-26.0798, -28.131) (-26.2516, -28.2931) (-26.7476, -28.4649) (-27.1074, -28.4649) knots 0 0 0 1 2 2 2
  line L83 (-27.1074, -28.4649) -> (-27.3829, -28.4649)
  line L84 (-27.3829, -28.4649) -> (-27.3829, -26.3871)
  spline S88 degree 2 poles (-27.3829, -26.3871) (-27.9048, -26.3871) (-28.4591, -26.9122) (-28.4591, -27.379) knots 0 0 0 1 2 2 2
  spline S89 degree 2 poles (-28.4591, -27.379) (-28.4591, -27.5443) (-28.3845, -27.8652) (-28.3262, -27.9948) knots 0 0 0 1 2 2 2
  spline S90 degree 2 poles (-28.3262, -27.9948) (-28.2614, -28.131) (-28.1479, -28.319) (-28.0961, -28.3806) knots 0 0 0 1 2 2 2
  line L85 (-28.0961, -28.3806) -> (-28.0961, -28.4098)
  line L86 (-28.0961, -28.4098) -> (-28.6471, -28.4098)
  spline S91 degree 2 poles (-28.6471, -28.4098) (-28.6828, -28.3222) (-28.7865, -28.0564) (-28.8157, -27.9527) knots 0 0 0 1 2 2 2
  spline S92 degree 2 poles (-28.8157, -27.9527) (-28.8578, -27.8068) (-28.8999, -27.567) (-28.8999, -27.3854) knots 0 0 0 1 2 2 2
  spline S93 degree 2 poles (-26.9972, -27.9722) (-26.793, -27.9657) (-26.4948, -27.8814) (-26.3943, -27.8004) knots 0 0 0 1 2 2 2
  spline S94 degree 2 poles (-26.3943, -27.8004) (-26.2808, -27.7128) (-26.1609, -27.4373) (-26.1609, -27.2331) knots 0 0 0 1 2 2 2
  spline S95 degree 2 poles (-26.1609, -27.2331) (-26.1609, -27.0321) (-26.2808, -26.7501) (-26.3975, -26.6334) knots 0 0 0 1 2 2 2
  spline S96 degree 2 poles (-26.3975, -26.6334) (-26.5174, -26.52) (-26.8059, -26.4033) (-26.9972, -26.3871) knots 0 0 0 1 2 2 2
  line L87 (-26.9972, -26.3871) -> (-26.9972, -27.9722)
  spline S97 degree 2 poles (-28.8999, -30.2801) (-28.8999, -29.5605) (-28.0928, -28.7696) (-27.3473, -28.7696) knots 0 0 0 1 2 2 2
  spline S98 degree 2 poles (-27.3473, -28.7696) (-26.6147, -28.7696) (-25.746, -29.5378) (-25.746, -30.1569) knots 0 0 0 1 2 2 2
  spline S99 degree 2 poles (-25.746, -30.1569) (-25.746, -30.4357) (-25.908, -30.8668) (-26.0798, -31.0256) knots 0 0 0 1 2 2 2
  spline S100 degree 2 poles (-26.0798, -31.0256) (-26.2516, -31.1877) (-26.7476, -31.3595) (-27.1074, -31.3595) knots 0 0 0 1 2 2 2
  line L88 (-27.1074, -31.3595) -> (-27.3829, -31.3595)
  line L89 (-27.3829, -31.3595) -> (-27.3829, -29.2817)
  spline S101 degree 2 poles (-27.3829, -29.2817) (-27.9048, -29.2817) (-28.4591, -29.8068) (-28.4591, -30.2736) knots 0 0 0 1 2 2 2
  spline S102 degree 2 poles (-28.4591, -30.2736) (-28.4591, -30.4389) (-28.3845, -30.7598) (-28.3262, -30.8895) knots 0 0 0 1 2 2 2
  spline S103 degree 2 poles (-28.3262, -30.8895) (-28.2614, -31.0256) (-28.1479, -31.2136) (-28.0961, -31.2752) knots 0 0 0 1 2 2 2
  line L90 (-28.0961, -31.2752) -> (-28.0961, -31.3044)
  line L91 (-28.0961, -31.3044) -> (-28.6471, -31.3044)
  spline S104 degree 2 poles (-28.6471, -31.3044) (-28.6828, -31.2169) (-28.7865, -30.9511) (-28.8157, -30.8474) knots 0 0 0 1 2 2 2
  spline S105 degree 2 poles (-28.8157, -30.8474) (-28.8578, -30.7015) (-28.8999, -30.4616) (-28.8999, -30.2801) knots 0 0 0 1 2 2 2
  spline S106 degree 2 poles (-26.9972, -30.8668) (-26.793, -30.8603) (-26.4948, -30.776) (-26.3943, -30.695) knots 0 0 0 1 2 2 2
  spline S107 degree 2 poles (-26.3943, -30.695) (-26.2808, -30.6075) (-26.1609, -30.332) (-26.1609, -30.1277) knots 0 0 0 1 2 2 2
  spline S108 degree 2 poles (-26.1609, -30.1277) (-26.1609, -29.9268) (-26.2808, -29.6448) (-26.3975, -29.5281) knots 0 0 0 1 2 2 2
  spline S109 degree 2 poles (-26.3975, -29.5281) (-26.5174, -29.4146) (-26.8059, -29.2979) (-26.9972, -29.2817) knots 0 0 0 1 2 2 2
  line L92 (-26.9972, -29.2817) -> (-26.9972, -30.8668)
  point P0 (0, 0)
  point P1 (-24.8059, 2.2745)
  dimension "d85" = 0.25
  dimension "d86" = 0.25
  constraints: 1 midpoint, 4 other
  measures "d85" distance between parallel lines of L4 L8
  measures "d86" distance from line of L9 point (-24.806, 2.274)
emboss "Emboss1" sketch "Sketch18" operation cut depth 1 direction (1, 0, 0)
equation "\"BendReliefWidth\" = Thickness"
equation "\"BendRadius\" = Thickness"
equation "\"BendReliefDepth\" = 0.5 * Thickness"
equation "\"CornerReliefSize\" = 4 * Thickness"
equation "\"MinimumRemnant\" = 2 * Thickness"
equation "\"TransitionRadius\" = BendRadius"
equation "\"JacobiRadiusSize\" = BendRadius"
equation "\"GapSize\" = Thickness"
equation "\"Thickness\" = 0.5"
body "Solid1"
